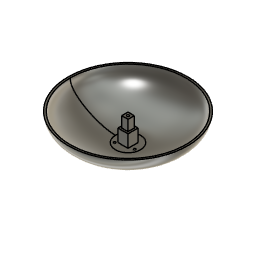
hub_roof_1 (Autodesk Fusion 360 design; units mm, degrees)
Autodesk Fusion 360 part; units mm, degrees
sketch "Sketch4" plane through (0, 0, 0) normal (0, 1, 0) x (1, 0, 0)
  spline S0 degree 5 poles (-20, 0) (-21.6536, 0) (-25.032, -0.1163) (-30.3134, -0.6396) (-37.7509, -2.0184) (-47.5071, -4.7949) (-57.4279, -8.5303) (-67.1391, -13.1315) (-76.1973, -18.5102) (-84.096, -24.5687) (-90.2992, -31.2112) (-93.4994, -36.932) (-94.7271, -41.4301) (-95, -44.5189) (-95, -46.0858) knots 0 0 0 0 0 0 0.1 0.2 0.3 0.4 0.5 0.6 0.7 0.8 0.9 1 1 1 1 1 1
  line L0 (-10, 0) -> (-30, 0)
  line L1 (-95, -36.0858) -> (-95, -56.0858)
  line L2 (-20, 0) -> (0, 0)
  line L3 (0, 0) -> (0, -3)
  spline S1 degree 3 poles (-20, -3) (-25.5966, -3) (-31.8408, -3.86) (-38.4727, -5.5163) (-46.4841, -7.517) (-55.0516, -10.6655) (-63.0384, -14.6677) (-71.1871, -18.751) (-78.7025, -23.7427) (-83.9452, -29.1422) (-87.2771, -32.5738) (-89.6623, -36.1401) (-90.918, -39.7495) (-91.6382, -41.8195) (-92, -43.9101) (-92, -46.0858) knots 0 0 0 0 0.213996 0.213996 0.213996 0.472505 0.472505 0.472505 0.736252 0.736252 0.736252 0.903871 0.903871 0.903871 1 1 1 1
  line L4 (-20, -3) -> (0, -3)
  line L5 (-95, -46.0858) -> (-92, -46.0858)
  point P0 (-70, -15)
  dimension "d30" = 20
  dimension "d45" = 3
  dimension "d46" = -3
  constraint coincident L2.end L3.start
  constraint perpendicular L2 L3
  measures "d30" distance of S0.start L2.end
  measures "d45" distance of L2.end L3.end
revolve "Revolve1" add sketch "Sketch4" angle 360 about axis through (0, 0, 1.75) along (0, 0, 1) makes body 1
sketch "Sketch5" plane through (0, 0, 3) normal (0, 0, 1) x (-1, 0, 0)
  line L0 (5, 5) -> (-5, 5)
  line L1 (-5, 5) -> (-5, -5)
  line L2 (-5, -5) -> (5, -5)
  line L3 (5, -5) -> (5, 5)
  line L4 (5, 5) -> (-5, -5) construction
  line L5 (-5, 5) -> (5, -5) construction
  line L6 (-8, 8) -> (-8, -8)
  line L7 (-8, -8) -> (8, -8)
  line L8 (8, -8) -> (8, 8)
  line L9 (8, 8) -> (-8, 8)
  circle A0 centre (0, 0) radius 20
  dimension "d33" = 10
  dimension "d34" = 10
  dimension "d35" = 3
  constraint horizontal L0
  constraint perpendicular L0 L1
  constraint parallel L0 L2
  constraint parallel L1 L3
  constraint coincident L4 A0.centre
  constraint coincident L5 A0.centre
  measures "d33" distance of L1.end L2.end
  measures "d34" distance of L0.end L1.end
extrude "Extrude2" add sketch "Sketch5" along normal blind 37 separate body contours L0 L1 L2 L3 makes body 2
sketch "Sketch6" plane through (0, 0, 40) normal (0, 0, 1) x (-1, 0, 0)
  circle A0 centre (0, 0) radius 2.05
  line L0 (5, -5) -> (5, 5)
  line L1 (5, 5) -> (-5, 5)
  line L2 (-5, 5) -> (-5, -5)
  line L3 (-5, -5) -> (5, -5)
  dimension "d16" = 4.1
  constraint coincident A0.centre origin
  measures "d16" diameter of A0
extrude "Extrude3" cut sketch "Sketch6" against normal blind 15 contours A0 bodies 2 1
sketch "Sketch7" plane through (0, 0, 0) normal (0, 0, -1) x (1, 0, 0)
  circle A0 centre (0, 0) radius 20
  circle A1 centre (-10.6066, 10.6066) radius 1.75
  circle A2 centre (-3.8823, -14.4889) radius 1.75
  circle A3 centre (14.4889, 3.8823) radius 1.75
  line L0 (0, 0) -> (-10.6066, 10.6066) construction
  dimension "d19" = 3.5
  dimension "d23" = 360
  dimension "d32" = 15
  constraint coincident A0.centre L0.start
  constraint coincident A1.centre L0.end
  measures "d19" diameter of A1
  measures "d32" distance of A0.centre A1.centre
extrude "Extrude4" cut sketch "Sketch7" against normal blind 15 contours A1 | A2 | A3 bodies 1 2
extrude "Extrude7" add sketch "Sketch5" along normal blind 20 contours L6 L7 L8 L9 bodies 1
sketch "Sketch9" plane through (0, 0, 3) normal (0, 0, 1) x (-1, 0, 0)
  line L0 (5, 5) -> (-5, 5)
  line L1 (-5, 5) -> (-5, -5)
  line L2 (-5, -5) -> (5, -5)
  line L3 (5, -5) -> (5, 5)
  circle A0 centre (0, 0) radius 1.75
  circle A1 centre (0, 0) radius 20
  circle A2 centre (3.8823, -14.4889) radius 1.75
  circle A3 centre (-14.4889, 3.8823) radius 1.75
  circle A4 centre (10.6066, 10.6066) radius 1.75
  line L4 (8, 8) -> (8, -8)
  line L5 (8, -8) -> (-8, -8)
  line L6 (-8, -8) -> (-8, 8)
  line L7 (-8, 8) -> (8, 8)
  dimension "d39" = 3.5
  constraint coincident A0.centre A1.centre
  measures "d39" diameter of A0
extrude "Extrude8" cut sketch "Sketch9" against normal blind 5 contours A0 bodies 1
extrude "Extrude9" cut sketch "Sketch9" along normal blind 10 contours A0 bodies 2
